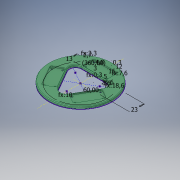
# Autodesk Inventor part: Stewart-Plate-inside
Saved by Autodesk Inventor 2018.2 (Build 222227000, 227)
## iProperties
Created: 2018-02-18
Part Number: Stewart-Plate-inside
Material: Generisch
Document SubType Name: Modeling
Designer: JochenAlt
Density: 1 g/cm^3
Appearance: Vorgabe
Author: JochenAlt
Autodesk Inventor part; units mm, degrees
ref_plane "YZ Plane" through (0, 0, 0) normal (1, 0, 0) x (0, 1, 0)
ref_plane "XZ Plane" through (0, 0, 0) normal (0, 1, 0) x (-1, 0, 0)
ref_plane "XY Plane" through (0, 0, 0) normal (0, 0, 1) x (1, 0, 0)
sketch "Skizze1" plane through (0, 0, 0) normal (0, 0, 1) x (1, 0, 0)
  line L0 (-11.2, 0) -> (11.2, 0) construction
  line L1 (-8, 36) -> (8, 36)
  line L2 (8, 36) -> (8, 33)
  line L3 (8, 33) -> (-8, 33)
  line L4 (-8, 33) -> (-8, 36)
  line L5 (1.5, 33) -> (-1.5, 33)
  line L6 (-1.5, 33) -> (-1.5, 28)
  line L7 (-1.5, 28) -> (1.5, 28)
  line L8 (1.5, 28) -> (1.5, 33)
  dimension "d10" = 3
  dimension "d14" = 16
  dimension "d23" = 5
  constraints: 16 end point, 4 parallel, 3 perpendicular, 2 horizontal, 1 point on line
  measures "d10" distance between parallel lines of L3 L1
  measures "d14" distance between parallel lines of L2 L4
  measures "d23" distance between parallel lines of L3 L7
extrude "Extrusion3" add sketch "Skizze1" against normal blind 7
fillet "Rundung1" radius 4 2 edges at (-8, 34.5, -7) (8, 34.5, -7)
sketch "Skizze2" plane through (-8, 36, 0) normal (0, 1, 0) x (1, 0, 0)
  circle A0 centre (3, 4) radius 1.1
  circle A1 centre (13, 4) radius 1.1
  line L0 (8, 0) -> (8, 7) construction
  line L1 (43, 0) -> (-27, 0) construction
  line L2 (-1.6221, 4) -> (19.0112, 4) construction
  line L3 (0, 7) -> (16, 7) construction
  line L4 (0, 0) -> (0, 7) projected
  point P0 (4, 7)
  point P1 (12, 7)
  point P2 (0, 3)
  dimension "d16" = 2.2
  dimension "d20" = 3
  dimension "d21" = 3
  constraints: 4 end point, 2 centre point, 1 equal radius, 1 horizontal, 1 midpoint, 1 point on line, 1 symmetric about line, 1 vertical
  measures "d16" diameter of A0
  measures "d20" distance between parallel lines of L3 L2
  measures "d21" distance from line of L4 A0.centre
extrude "Extrusion4" cut sketch "Skizze2" against normal up to next
chamfer "Fase1" distance 5 distance2 7 1 edges at (0, 28, -7) measured on face at (0, 28.5, -7)
pattern_circular "Runde Anordnung1" count 3 over 360 about axis through (0, 0, -10) along (0, 0, 1) of "Extrusion3", "Extrusion4", "Fase1", "Rundung1"
sketch "Skizze3" plane through (0, 0, 0) normal (0, 0, 1) x (1, 0, 0)
  line L0 (0, 69.6967) -> (0, -69.6967) construction
  circle A0 centre (0, 0) radius 39 construction
  circle A1 centre (0, 0) radius 51.0665
  line L1 (19.75, 21.2) -> (-19.399, 21.2)
  line L2 (-28.0592, 6.2) -> (-8.6603, -27.4)
  line L3 (28.2347, 6.504) -> (8.6603, -27.4)
  line L4 (-28.1902, 15.9659) -> (18.4475, -10.448) construction
  line L5 (36.7195, 21.2) -> (-18.3597, -10.6) construction
  arc A2 (28.2347, 6.504) -> (19.75, 21.2) centre (19.75, 11.4027) ccw
  arc A3 (-19.399, 21.2) -> (-28.0592, 6.2) centre (-19.399, 11.2) ccw
  arc A4 (-8.6603, -27.4) -> (8.6603, -27.4) centre (0, -22.4) ccw
  line L6 (0.15, 49.6) -> (12.15, 49.6) construction
  line L7 (12.15, 49.6) -> (12.15, 23) construction
  line L8 (12.15, 23) -> (0.15, 23) construction
  line L9 (0.15, 23) -> (0.15, 49.6) construction
  line L10 (-0.15, 49.6) -> (-12.15, 49.6) construction
  line L11 (-12.15, 49.6) -> (-12.15, 23) construction
  line L12 (-12.15, 23) -> (-0.15, 23) construction
  line L13 (-0.15, 23) -> (-0.15, 49.6) construction
  line L14 (-17.45, 41.3) -> (17.45, 41.3)
  line L15 (19.75, 39) -> (19.75, 25)
  line L16 (17.45, 22.7) -> (-17.45, 22.7)
  line L17 (-19.75, 25) -> (-19.75, 39)
  arc A5 (-17.45, 41.3) -> (-19.75, 39) centre (-17.45, 39) ccw
  arc A6 (-19.75, 25) -> (-17.45, 22.7) centre (-17.45, 25) ccw
  arc A7 (17.45, 22.7) -> (19.75, 25) centre (17.45, 25) ccw
  arc A8 (19.75, 39) -> (17.45, 41.3) centre (17.45, 39) ccw
  circle A9 centre (-16.95, 38.65) radius 1.35
  circle A10 centre (-16.95, 25.65) radius 1.35
  circle A11 centre (16.95, 38.65) radius 1.35
  circle A12 centre (16.95, 25.65) radius 1.35
  line L18 (-19.75, 32.15) -> (19.75, 32.15) construction
  line L19 (-16.95, 38.65) -> (-16.95, 25.65) construction
  arc A13 (-27.0418, -35.7621) -> (-23.9, -36.604) centre (-25.05, -34.6121) ccw
  line L20 (-11.7756, -29.604) -> (-23.9, -36.604)
  circle A14 centre (-24.9969, -34.0041) radius 1.35
  line L21 (-27.0418, -35.7621) -> (-44.4918, -5.5379)
  circle A15 centre (-13.7386, -27.5041) radius 1.35
  arc A16 (-11.7756, -29.604) -> (-10.9338, -26.4621) centre (-12.9256, -27.6121) ccw
  line L22 (-28.3838, 3.7621) -> (-10.9338, -26.4621)
  arc A17 (-28.3838, 3.7621) -> (-31.5256, 4.604) centre (-30.3756, 2.6121) ccw
  circle A18 centre (-30.6886, 1.8541) radius 1.35
  arc A19 (-43.65, -2.396) -> (-44.4918, -5.5379) centre (-42.5, -4.3879) ccw
  circle A20 centre (-41.9469, -4.6459) radius 1.35
  line L23 (-43.65, -2.396) -> (-31.5256, 4.604)
  arc A21 (44.4918, -5.5379) -> (43.65, -2.396) centre (42.5, -4.3879) ccw
  line L24 (31.5256, 4.604) -> (43.65, -2.396)
  circle A22 centre (41.9469, -4.6459) radius 1.35
  line L25 (44.4918, -5.5379) -> (27.0418, -35.7621)
  circle A23 centre (30.6886, 1.8541) radius 1.35
  arc A24 (31.5256, 4.604) -> (28.3838, 3.7621) centre (30.3756, 2.6121) ccw
  line L26 (10.9338, -26.4621) -> (28.3838, 3.7621)
  arc A25 (10.9338, -26.4621) -> (11.7756, -29.604) centre (12.9256, -27.6121) ccw
  circle A26 centre (13.7386, -27.5041) radius 1.35
  arc A27 (23.9, -36.604) -> (27.0418, -35.7621) centre (25.05, -34.6121) ccw
  circle A28 centre (24.9969, -34.0041) radius 1.35
  line L27 (23.9, -36.604) -> (11.7756, -29.604)
  point P0 (-36.7195, 21.2)
  point P1 (0, -42.4)
  point P2 (-17.9677, -33.179)
  point P3 (-37.7177, 1.029)
  point P4 (37.7177, 1.029)
  point P5 (17.9677, -33.179)
  dimension "d140" = 60
  dimension "d144" = 10
  dimension "d146" = 0.3
  dimension "d147" = 26.6
  dimension "d148" = 12
  dimension "d150" = 0.3
  dimension "d151" = 18.6
  dimension "d152" = 2.3
  dimension "d153" = 13
  dimension "d154" = 7.6
  dimension "d155" = 4.8
  dimension "d158" = 360
  dimension "d160" = 1.5
  dimension "d161" = 2.7
  dimension "d164" = 23
  constraints: 54 end point, 31 point on circle, 27 centre point, 16 point on line, 14 tangent, 7 equal radius, 6 parallel, 4 perpendicular, 3 horizontal, 2 collinear, 2 midpoint, 2 symmetric about line, 1 coincident, 1 vertical, 100 other
  measures "d140" angle of L3 L1
  measures "d144" radius of A4
  measures "d146" distance between parallel lines of L9 L13
  measures "d147" distance between parallel lines of L8 L6
  measures "d148" distance between parallel lines of L7 L9
  measures "d150" distance between parallel lines of L16 L8
  measures "d151" distance between parallel lines of L16 L14
  measures "d152" radius of A5
  measures "d153" distance of L19.end L19.start
  measures "d154" distance between parallel lines of L15 L7
  measures "d155" distance between parallel lines of L11 L19
  measures "d160" distance between parallel lines of L1 L16
  measures "d161" diameter of A9
  measures "d164" distance from line of point (0, 0) L8
extrude "Extrusion11" add sketch "Skizze3" along normal blind 4 contours A1 | A2 L3 A4 L2 A3 L1 | L14 A8 L15 A7 L16 A6 L17 A5 | A9 | A10 | A11 | A12 | L21 A19 L23 A17 L22 A16 L20 A13 | A14 | A15 | A18 | A20 | L25 A27 L27 A25 L26 A24 L24 A21 | A22 | A23 | A26 | A28
extrude "Extrusion9" cut sketch "Skizze3" along normal blind 4 contours A2 L3 A4 L2 A3 L1 | L14 A8 L15 A7 L16 A6 L17 A5 | A9 | A10 | A11 | A12 | L21 A19 L23 A17 L22 A16 L20 A13 | A14 | A15 | A18 | A20 | L25 A27 L27 A25 L26 A24 L24 A21 | A22 | A23 | A26 | A28
extrude "Extrusion6" add sketch "Skizze3" along normal blind 2 contours L14 A8 L15 A7 L16 A6 L17 A5 | L21 A19 L23 A17 L22 A16 L20 A13 | L25 A27 L27 A25 L26 A24 L24 A21
fillet "Rundung4" radius 1 14 edges at (-51.0665, 0, 4) (0.1755, 21.2, 4) (28.2347, 16.3013, 4) (18.4475, -10.448, 4) (0, -32.4, 4) (-18.3597, -10.6, 4) (-28.0592, 16.2, 4) (-18.3597, -10.6, 0) (0, -32.4, 0) (18.4475, -10.448, 0) (28.2347, 16.3013, 0) (0.1755, 21.2, 0) (-28.0592, 16.2, 0) (-51.0665, 0, 0)
equation "\"d21\" = d20"
